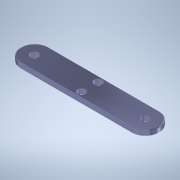
# Autodesk Inventor part: steering_top_plane
Saved by Autodesk Inventor 2020 (Build 240168000, 168)
## iProperties
Created: 2015-12-07
Part Number: steering_top_plane
Material: Acero, aleación
Document SubType Name: Modeling
Designer: MIGUEL ANGEL
Density: 7.73 g/cm^3
Appearance: Cromo - Azul Pulido
Author: MIGUEL ANGEL
Autodesk Inventor part; units mm, degrees
ref_plane "YZ Plane" through (0, 0, 0) normal (1, 0, 0) x (0, 1, 0)
ref_plane "XZ Plane" through (0, 0, 0) normal (0, 1, 0) x (-1, 0, 0)
ref_plane "XY Plane" through (0, 0, 0) normal (0, 0, 1) x (1, 0, 0)
sketch "Boceto1" plane through (0, 0, 0) normal (0, 0, 1) x (1, 0, 0)
  line L0 (-40, 10) -> (40, 10)
  arc A0 (40, -10) -> (40, 10) centre (40, 0) ccw
  line L1 (40, -10) -> (-40, -10)
  arc A1 (-40, 10) -> (-40, -10) centre (-40, 0) ccw
  circle A2 centre (-40, 0) radius 3
  circle A3 centre (40, 0) radius 3
  circle A4 centre (0, 6) radius 3
  circle A5 centre (0, -6) radius 3
  point P0 (0, 0)
  point P1 (0, 10)
  point P2 (50, 0)
  dimension "d0" = 10
  dimension "d1" = 80
  dimension "d2" = 6
  dimension "d3" = 4
  dimension "d4" = 4
  constraints: 6 centre point, 5 point on circle, 4 end point, 4 tangent, 3 equal radius, 2 coincident, 1 horizontal, 1 horizontal alignment, 1 midpoint, 1 parallel, 1 vertical alignment
  measures "d0" radius of A0
  measures "d1" distance of L0.start L0.end
  measures "d2" diameter of A2
  measures "d3" distance of point (0, 10) A4.centre
  measures "d4" distance from line of L1 A5.centre
extrude "Extrusión1" add sketch "Boceto1" along normal blind 4
chamfer "Chaflán1" distance 0.5 angle 45 8 edges at (50, 0, 0) (0, -10, 0) (-50, 0, 0) (0, 10, 0) (50, 0, 4) (0, 10, 4) (-50, 0, 4) (0, -10, 4)
equation "\"d4\" = d3"
